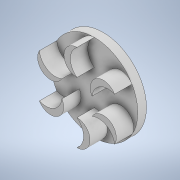
# Autodesk Inventor part: 20220627_fan
Saved by Autodesk Inventor 2020 (Build 240168000, 168)
## iProperties
Created: 2022-06-27
Part Number: 20220627_fan
Material: 一般
Document SubType Name: Modeling
Designer: Naggy
Density: 1 g/cm^3
Appearance: 既定
Author: Naggy
Autodesk Inventor part; units mm, degrees
ref_plane "YZ Plane" through (0, 0, 0) normal (1, 0, 0) x (0, 1, 0)
ref_plane "XZ Plane" through (0, 0, 0) normal (0, 1, 0) x (-1, 0, 0)
ref_plane "XY Plane" through (0, 0, 0) normal (0, 0, 1) x (1, 0, 0)
sketch "スケッチ1" plane through (0, 0, 0) normal (0, 0, 1) x (1, 0, 0)
  circle A0 centre (0, 0) radius 25
  dimension "d0" = 50
  constraints: 1 centre point, 1 coincident
  measures "d0" diameter of A0
extrude "押し出し1" add sketch "スケッチ1" along normal blind 5
sketch "スケッチ2" plane through (0, 0, 5) normal (0, 0, 1) x (1, 0, 0)
  circle A0 centre (0, 0) radius 10
  circle A1 centre (0, 0) radius 25 projected
  arc A2 (0, 25) -> (0, 10) centre (0, 17.5) ccw
  arc A3 (0, 25) -> (0, 10) centre (5.5238, 17.5) ccw
  arc A4 (-21.6506, 12.5) -> (-8.6603, 5) centre (-12.3935, 13.5338) ccw
  arc A5 (-21.6506, 12.5) -> (-8.6603, 5) centre (-15.1554, 8.75) ccw
  arc A6 (-21.6506, -12.5) -> (-8.6603, -5) centre (-17.9174, -3.9662) ccw
  arc A7 (-21.6506, -12.5) -> (-8.6603, -5) centre (-15.1554, -8.75) ccw
  arc A8 (0, -25) -> (0, -10) centre (-5.5238, -17.5) ccw
  arc A9 (0, -25) -> (0, -10) centre (0, -17.5) ccw
  arc A10 (21.6506, -12.5) -> (8.6603, -5) centre (12.3935, -13.5338) ccw
  arc A11 (21.6506, -12.5) -> (8.6603, -5) centre (15.1554, -8.75) ccw
  arc A12 (21.6506, 12.5) -> (8.6603, 5) centre (17.9174, 3.9662) ccw
  arc A13 (21.6506, 12.5) -> (8.6603, 5) centre (15.1554, 8.75) ccw
  dimension "d3" = 20
  dimension "d6" = 360
  constraints: 24 point on circle, 12 centre point, 2 vertical alignment, 1 coincident, 41 other
extrude "押し出し2" add sketch "スケッチ2" along normal blind 10 contours A13 A12 | A11 A10 | A2 A3 | A9 A8 | A5 A4 | A7 A6
sketch "スケッチ3" plane through (0, 0, 5) normal (0, 0, 1) x (1, 0, 0)
  point P0 (0, 0)
hole "穴1" at (0, 0, 5) direction (0, 0, -1) diameter 1.8 depth 8.8 tip angle 118
